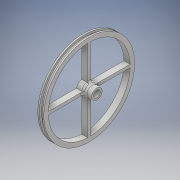
# Autodesk Inventor part: mtv_brakeWheel(61mm)_1-14
Saved by Autodesk Inventor 2018 (Build 220112000, 112)
## iProperties
Created: 2019-01-15
Part Number: mtv_brakeWheel(61mm)_1-14
Material: Generic
Document SubType Name: Modeling
Designer: aditya
Density: 1 g/cm^3
Appearance: Default
Author: aditya
## iProperties of the stored document mtv_brakeWheel(61mm)_1-14_3DPrint.ipt
Created: 2019-01-15
Part Number: mtv_brakeWheel(61mm)_1-14_3DPrint
Material: Generic
Document SubType Name: Modeling
Designer: aditya
Density: 1 g/cm^3
Appearance: Default
Author: aditya
Autodesk Inventor part; units mm, degrees
ref_plane "YZ Plane" through (0, 0, 0) normal (1, 0, 0) x (0, 1, 0)
ref_plane "XZ Plane" through (0, 0, 0) normal (0, 1, 0) x (-1, 0, 0)
ref_plane "XY Plane" through (0, 0, 0) normal (0, 0, 1) x (1, 0, 0)
sketch "Sketch1" plane through (0, 0, 0) normal (1, 0, 0) x (0, 1, 0)
  circle A0 centre (0, 0) radius 28.5
  dimension "d0" = 57
  constraints: 1 centre point, 1 coincident
  measures "d0" diameter of A0
extrude "Extrusion1" add sketch "Sketch1" along normal blind 2
sketch "Sketch2" plane through (2, 0, 0) normal (1, 0, 0) x (0, 0, -1)
  circle A0 centre (0, 0) radius 30
  dimension "d3" = 60
  constraints: 1 centre point, 1 coincident
  measures "d3" diameter of A0
extrude "Extrusion2" add sketch "Sketch2" along normal blind 1
sketch "Sketch3" plane through (0, 0, 0) normal (-1, 0, 0) x (0, 0, 1)
  circle A0 centre (0, 0) radius 30
  dimension "d6" = 60
  constraints: 1 centre point, 1 coincident
  measures "d6" diameter of A0
extrude "Extrusion3" add sketch "Sketch3" along normal blind 1
sketch "Sketch4" plane through (-1, 0, 0) normal (-1, 0, 0) x (0, 0, 1)
  circle A0 centre (0, 0) radius 27
  dimension "d9" = 54
  constraints: 1 centre point, 1 coincident
  measures "d9" diameter of A0
extrude "Extrusion4" cut sketch "Sketch4" against normal blind 10
sketch "Sketch5" plane through (-1, 0, 0) normal (-1, 0, 0) x (0, 0, 1)
  circle A0 centre (0, 0) radius 2.125
  circle A1 centre (0, 0) radius 3.25
  dimension "d12" = 4.25
  dimension "d13" = 6.5
  constraints: 2 centre point, 2 coincident
  measures "d12" diameter of A0
  measures "d13" diameter of A1
extrude "Extrusion5" add sketch "Sketch5" against normal blind 4
sketch "Sketch6" plane through (-1, 0, 0) normal (-1, 0, 0) x (0, 0, 1)
  line L0 (-2.9572, 0) -> (-2.9572, 1) construction
  line L1 (-2.9572, 1) -> (-2.9572, -1) construction
  line L2 (-2.9572, 1) -> (-27.9528, 1)
  line L3 (-27.9528, 1) -> (-27.9528, -1)
  line L4 (-27.9528, -1) -> (-2.9572, -1)
  line L5 (-2.9572, -1) -> (-2.9572, 1)
  point P0 (0, 0)
  dimension "d16" = 1
  dimension "d17" = 2
  constraints: 12 end point, 2 parallel, 1 horizontal, 1 perpendicular, 1 point on line, 1 vertical
  measures "d16" distance of L0.start L0.end
  measures "d17" distance of L0.end L1.end
extrude "Extrusion6" add sketch "Sketch6" against normal blind 4
pattern_circular "Circular Pattern1" count 4 over 360 about axis through (-1, 0, 0) along (1, 0, 0) of "Extrusion6"
sketch "Sketch7" plane through (3, 0, 0) normal (1, 0, 0) x (0, 0, -1)
  circle A0 centre (0, 0) radius 2.125
  circle A1 centre (0, 0) radius 3.25
  constraints: 2 centre point, 2 coincident
extrude "Extrusion7" add sketch "Sketch7" along normal blind 5
sketch "Sketch8" plane through (8, 0, 0) normal (1, 0, 0) x (0, 0, -1)
  circle A0 centre (0, 0) radius 4.5
  circle A1 centre (0, 0) radius 2.125
  circle A2 centre (0, 0) radius 2.125
  dimension "d25" = 9
  dimension "d26" = 4.25
  constraints: 3 centre point, 3 coincident
  measures "d25" diameter of A0
  measures "d26" diameter of A2
extrude "Extrusion8" add sketch "Sketch8" against normal blind 9
sketch "Sketch9" plane through (8, 0, 0) normal (1, 0, 0) x (0, 0, -1)
  circle A0 centre (0, 0) radius 2.25
  circle A1 centre (0, 0) radius 4.5
  circle A2 centre (0, 0) radius 3.5
  dimension "d29" = 4.5
  dimension "d30" = 7
  constraints: 3 centre point, 3 coincident
  measures "d29" diameter of A0
  measures "d30" diameter of A2
extrude "Extrusion9" cut sketch "Sketch9" against normal blind 5 contours A1
sketch "Sketch10" plane through (8, 0, 0) normal (1, 0, 0) x (0, 0, -1)
  circle A0 centre (0, 0) radius 2.25
  dimension "d33" = 4.5
  constraints: 1 centre point, 1 coincident
  measures "d33" diameter of A0
extrude "Extrusion10" cut sketch "Sketch10" against normal blind 5000
fillet "Fillet1" radius 2 1 edges at (3, 0, 3.5)
fillet "Fillet2" radius 2 4 edges at (3.2679, 3.182, 3.182) (3.2679, -3.182, 3.182) (3.2679, 3.182, -3.182) (3.2679, -3.182, -3.182)
body "Solid1"
